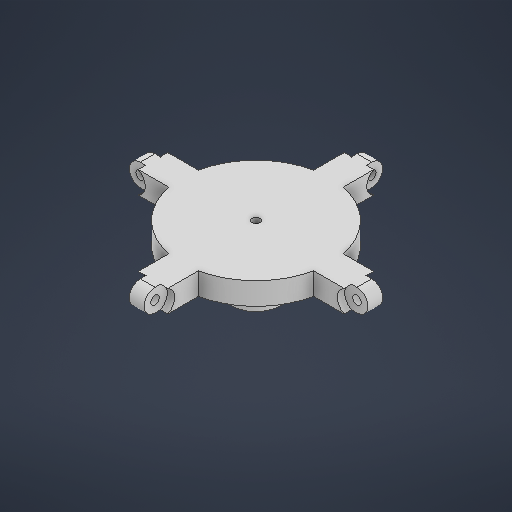
# Autodesk Inventor part: SujeccionHelices
Saved by Autodesk Inventor 2026.1 (Build 301233000, 233)
## iProperties
Created: 2025-11-10
Part Number: SujeccionHelices
Material: Genérico
Document SubType Name: Modeling
Designer: vickh
Density: 1 g/cm^3
Appearance: Valor por defecto
Author: vickh
Autodesk Inventor part; units mm, degrees
ref_plane "YZ Plane" through (0, 0, 0) normal (1, 0, 0) x (0, 1, 0)
ref_plane "XZ Plane" through (0, 0, 0) normal (0, 1, 0) x (-1, 0, 0)
ref_plane "XY Plane" through (0, 0, 0) normal (0, 0, 1) x (1, 0, 0)
sketch "Boceto3" plane through (0, 0, 0) normal (0, 1, 0) x (-1, 0, 0)
  line L0 (-50, 50) -> (50, 50) construction
  line L1 (50, 50) -> (50, -50) construction
  line L2 (50, -50) -> (-50, -50) construction
  line L3 (-50, -50) -> (-50, 50) construction
  line L4 (-50, 50) -> (50, -50) construction
  line L5 (50, 50) -> (-50, -50) construction
  circle A0 centre (0, 0) radius 10
  dimension "d5" = 100
  dimension "d6" = 100
  dimension "d7" = 20
  constraints: 12 end point, 2 midpoint, 2 parallel, 1 centre point, 1 coincident, 1 horizontal, 1 perpendicular
  measures "d5" distance of L1.end L2.end
  measures "d6" distance of L0.end L1.end
  measures "d7" diameter of A0
extrude "Extrusión2" add sketch "Boceto3" along normal blind 16
sketch "Boceto4" plane through (0, 16, 0) normal (0, 1, 0) x (1, 0, 0)
  line L0 (-48.5, -6) -> (-29.3939, -6)
  line L1 (-29.3939, 6) -> (-48.5, 6)
  line L2 (-48.5, 6) -> (-48.5, -6)
  line L3 (-48.5, -6) -> (-29.3939, 6) construction
  line L4 (-29.3939, -6) -> (-48.5, 6) construction
  line L5 (-73.8268, 0) -> (57.9613, 0) construction
  line L6 (-6, -29.3939) -> (-6, -48.5)
  line L7 (-6, -48.5) -> (6, -48.5)
  line L8 (6, -48.5) -> (6, -29.3939)
  line L9 (29.3939, -6) -> (48.5, -6)
  line L10 (48.5, -6) -> (48.5, 6)
  line L11 (48.5, 6) -> (29.3939, 6)
  line L12 (6, 29.3939) -> (6, 48.5)
  line L13 (6, 48.5) -> (-6, 48.5)
  line L14 (-6, 48.5) -> (-6, 29.3939)
  arc A0 (29.3939, 6) -> (6, 29.3939) centre (0, 0) ccw
  arc A1 (-6, 29.3939) -> (-29.3939, 6) centre (0, 0) ccw
  arc A2 (-29.3939, -6) -> (-6, -29.3939) centre (0, 0) ccw
  arc A3 (6, -29.3939) -> (29.3939, -6) centre (0, 0) ccw
  point P0 (-38.9469, 0)
  point P1 (-38.9469, 0)
  point P2 (-48.5, 0)
  point P3 (-38.9469, -6)
  point P4 (0, -48.5)
  point P5 (6, -38.9469)
  point P6 (48.5, 0)
  point P7 (38.9469, 6)
  point P8 (0, 48.5)
  point P9 (-6, 38.9469)
  dimension "d15" = 48.5
  dimension "d16" = 12
  dimension "d19" = 360
  dimension "d21" = 30
  constraints: 30 end point, 8 point on circle, 5 midpoint, 4 centre point, 2 horizontal, 2 point on line, 1 coincident, 1 parallel, 1 vertical, 37 other
  measures "d15" distance of point (0, 0) point (-48.5, 0)
  measures "d16" distance from line of point (-38.947, -6) L1
  measures "d21" radius of A0
extrude "Extrusión3" add sketch "Boceto4" along normal blind 9
sketch "Boceto7" plane through (0, 0, 0) normal (0, -1, 0) x (1, 0, 0)
  circle A0 centre (0, 0) radius 3.45
  dimension "d26" = 6.9
  constraints: 1 centre point, 1 coincident
  measures "d26" diameter of A0
extrude "Extrusión4" cut sketch "Boceto7" against normal blind 3.5
fillet "Empalme1" radius 4.5 8 edges at (0, 16, -48.5) (0, 25, -48.5) (48.5, 16, 0) (48.5, 25, 0) (0, 16, 48.5) (0, 25, 48.5) (-48.5, 16, 0) (-48.5, 25, 0)
sketch "Boceto9" plane through (-6, 16, 29.3939) normal (-1, 0, 0) x (0, 0, 1)
  line L0 (0, 0) -> (-23.3939, 0) projected
  line L1 (0, 0) -> (19.1061, 0) construction
  line L2 (19.1061, 0) -> (19.1061, 9) construction
  line L3 (19.1061, 9) -> (0, 9) construction
  line L4 (0, 9) -> (0, 0) construction
  arc A0 (14.6061, 0) -> (14.6061, 9) centre (14.6061, 4.5) ccw construction
  line L5 (0, 9) -> (14.6061, 9) construction
  line L6 (19.1061, 9) -> (0, 0) construction
  line L7 (0, 9) -> (19.1061, 0) construction
  line L8 (0, 0) -> (0, 9) construction
  line L9 (0, 4.5) -> (19.1061, 4.5) construction
  circle A1 centre (14.6061, 4.5) radius 1.75
  point P0 (-29.3939, -16)
  dimension "d31" = 3.5
  constraints: 14 end point, 2 parallel, 1 centre point, 1 coincident, 1 collinear, 1 horizontal, 1 midpoint, 1 perpendicular, 1 point on circle, 1 tangent
  measures "d31" diameter of A1
sketch "Boceto13" plane through (0, 25, 0) normal (0, 1, 0) x (1, 0, 0)
  circle A0 centre (0, 0) radius 3.45 projected
  line L0 (-44, -44) -> (44, -44)
  line L1 (44, -44) -> (44, 44)
  line L2 (44, 44) -> (-44, 44)
  line L3 (-44, 44) -> (-44, -44)
  line L4 (-44, -44) -> (44, 44) construction
  line L5 (44, -44) -> (-44, 44) construction
  line L6 (-44, -6) -> (-44, 6) projected
  line L7 (-6, 44) -> (6, 44) projected
  constraints: 12 end point, 2 collinear, 2 midpoint, 2 parallel, 1 horizontal, 1 perpendicular
sweep "Barrido1" cut profiles "Boceto9" path "Boceto13" path curves L3 L0 L1 L2
sketch "Boceto15" plane through (-29.3939, 16, 6) normal (0, 0, 1) x (1, 0, 0)
  circle A0 centre (-14.6061, 4.5) radius 1.75 projected
  circle A1 centre (-14.6061, 4.5) radius 5
  circle A2 centre (73.3939, 4.5) radius 1.75 projected
  circle A3 centre (73.3939, 4.5) radius 5
  point P0 (29.3939, -16)
  dimension "d47" = 10
  dimension "d54" = 10
  constraints: 2 centre point, 2 coincident
  measures "d47" diameter of A1
  measures "d54" diameter of A3
extrude "Extrusión9" cut sketch "Boceto15" against normal blind 3
sketch "Boceto16" plane through (-29.3939, 16, -6) normal (0, 0, -1) x (-1, 0, 0)
  circle A0 centre (14.6061, 4.5) radius 1.75 projected
  circle A1 centre (14.6061, 4.5) radius 5
  circle A2 centre (-73.3939, 4.5) radius 1.75 projected
  circle A3 centre (-73.3939, 4.5) radius 5
  point P0 (-29.3939, -16)
  dimension "d50" = 10
  dimension "d51" = 10
  constraints: 2 centre point, 2 coincident
  measures "d50" diameter of A1
  measures "d51" diameter of A3
extrude "Extrusión10" cut sketch "Boceto16" against normal blind 3 contours A1 | A2 | A3
sketch "Boceto17" plane through (-6, 16, 29.3939) normal (-1, 0, 0) x (0, 0, 1)
  circle A0 centre (14.6061, 4.5) radius 1.75 projected
  circle A1 centre (-73.3939, 4.5) radius 1.75 projected
  circle A2 centre (-73.3939, 4.5) radius 5
  circle A3 centre (14.6061, 4.5) radius 5
  point P0 (-29.3939, -16)
  dimension "d55" = 10
  dimension "d56" = 10
  constraints: 2 centre point, 2 coincident
  measures "d55" diameter of A2
  measures "d56" diameter of A3
extrude "Extrusión11" cut sketch "Boceto17" against normal blind 3
sketch "Boceto18" plane through (6, 16, 29.3939) normal (1, 0, 0) x (0, 0, -1)
  circle A0 centre (-14.6061, 4.5) radius 1.75 projected
  circle A1 centre (73.3939, 4.5) radius 1.75 projected
  circle A2 centre (-14.6061, 4.5) radius 5
  circle A3 centre (73.3939, 4.5) radius 5
  point P0 (29.3939, -16)
  dimension "d59" = 10
  dimension "d60" = 10
  constraints: 2 centre point, 2 coincident
  measures "d59" diameter of A2
  measures "d60" diameter of A3
extrude "Extrusión12" cut sketch "Boceto18" against normal blind 3
sketch "Boceto19" plane through (0, 25, 0) normal (0, 1, 0) x (1, 0, 0)
  circle A0 centre (0, 0) radius 1.6
  dimension "d63" = 3.2
  constraints: 1 centre point, 1 coincident
  measures "d63" diameter of A0
extrude "Extrusión13" cut sketch "Boceto19" against normal blind 20
